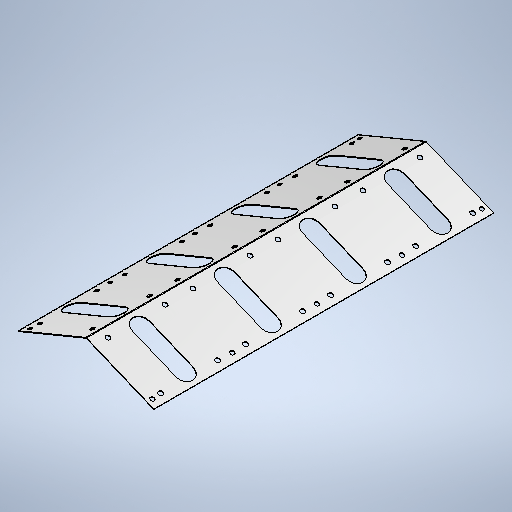
# Autodesk Inventor part: DMF 01 11 cylinder sheet cap v2.1
Saved by Autodesk Inventor 2026.2 (Build 302298010, 298A)
## iProperties
Created: 2024-04-28
Part Number: DMF 01 11 cylinder sheet cap v2.1
Material: Stainless Steel AISI 304
Document SubType Name: Sheet Metal
Designer: pokla
Density: 8 g/cm^3
Appearance: Chrome - Satin
Sheet Metal Rule: Default
Sheet Metal Width: 423,788 mm
Sheet Metal Length: 983,000 mm
Sheet Metal Area: 416583,808 mm^2
Flat Pattern Width: 42.3788 cm
Flat Pattern Length: 98.3 cm
Flat Pattern Area: 4165.84 cm^2
Stock Number: Барабан_Лист_Крышка
d192: 145,000 mm
d193: 50,000 mm
Author: pokla
Autodesk Inventor part; units mm, degrees
ref_plane "YZ Plane" through (0, 0, 0) normal (1, 0, 0) x (0, 1, 0)
ref_plane "XZ Plane" through (0, 0, 0) normal (0, 1, 0) x (-1, 0, 0)
ref_plane "XY Plane" through (0, 0, 0) normal (0, 0, 1) x (1, 0, 0)
sketch "Sketch1" plane through (0, 0, 0) normal (0, 0, 1) x (1, 0, 0)
  line L0 (-197.081968, 197.081968) -> (0, 278.715992) construction
  line L1 (0, 278.715992) -> (197.081968, 197.081968) construction
  line L2 (197.081968, 197.081968) -> (278.715992, 0) construction
  line L3 (278.715992, 0) -> (197.081968, -197.081968) construction
  line L4 (197.081968, -197.081968) -> (0, -278.715992) construction
  line L5 (0, -278.715992) -> (-197.081968, -197.081968) construction
  line L6 (-197.081968, -197.081968) -> (-278.715992, 0) construction
  line L7 (-278.715992, 0) -> (-197.081968, 197.081968) construction
  line L8 (1.530734, 278.081941) -> (196.250476, 197.426383)
  line L9 (-1.530734, 278.081941) -> (-196.250476, 197.426383)
  arc A0 (1.530734, 278.081941) -> (-1.530734, 278.081941) centre (0, 274.386423) ccw
  point P0 (0, 0)
  point P1 (0, 0)
  dimension "d46" = 515
  dimension "d47" = 0.9
  dimension "d48" = 4
  measures "d46" distance between parallel lines of L7 L3
  measures "d47" distance of L0.start L9.end
  measures "d48" radius of A0
contour flange "Contour Flange2" sketch "Sketch1" thickness 2 bend radius 2 width 983 along (0, 0, -1) mid plane no both sides no wall seen from (98.890605, 237.754162, 0) lies toward (-0.3826834, -0.9238795, 0) curves L8 A0 L9
bend "Bend4"
corner "Corner4"
sketch "Sketch14" plane through (1.530734, 278.081941, 0) normal (0.3826834, 0.9238795, 0) x (0.9238795, -0.3826834, 0)
  line L0 (173.881565, 148) -> (173.881565, 98) construction
  line L1 (173.881565, 98) -> (36.881565, 98)
  line L2 (36.881565, 98) -> (36.881565, 148) construction
  line L3 (36.881565, 148) -> (173.881565, 148)
  circle A0 centre (187.881565, 205.5) radius 6.5
  circle A1 centre (22.881565, 205.5) radius 6.5
  line L4 (105.381565, 98) -> (105.381565, 148) construction
  line L5 (210.76313, 0) -> (0, 0)
  line L6 (105.381565, 123) -> (173.881565, 123) construction
  circle A2 centre (22.881565, 40.5) radius 6.5
  circle A3 centre (187.881565, 40.5) radius 6.5
  arc A4 (173.881565, 98) -> (173.881565, 148) centre (173.881565, 123) ccw
  arc A5 (36.881565, 148) -> (36.881565, 98) centre (36.881565, 123) ccw
  point P0 (105.381565, 0)
  dimension "d163" = 13
  dimension "d164" = 137
  dimension "d165" = 50
  dimension "d167" = 165
  dimension "d171" = 98
  dimension "d181" = 165
  constraints: 12 end point, 6 centre point, 5 midpoint, 4 point on circle, 4 tangent, 2 parallel, 1 perpendicular, 1 vertical alignment, 3 other
  measures "d163" diameter of A0
  measures "d164" distance of L2.end L0.start
  measures "d165" distance of L0.start L0.end
  measures "d167" distance of A1.centre A0.centre
  measures "d171" distance between parallel lines of L5 L1
  measures "d181" distance of A1.centre A2.centre
extrude "Cut2" cut sketch "Sketch14" against normal through all
pattern_linear "Rectangular Pattern7" count 4 spacing 246 along (0, 0, -1) of "Cut2"
pattern_circular "Circular Pattern2" count 2 over 45 about axis through (0, 0, -10) along (0, 0, 1) of "Cut2", "Rectangular Pattern7"
sketch "Sketch16" plane through (0.765367, 276.234182, -983) normal (-0.3826834, -0.9238795, 0) x (0.9238795, -0.3826834, 0)
  circle A0 centre (189.76313, 968) radius 6
  line L0 (189.76313, 968) -> (189.76313, 15) construction
  circle A1 centre (189.76313, 15) radius 6
  circle A2 centre (189.76313, 246.5) radius 6
  circle A3 centre (189.76313, 491.5) radius 6
  circle A4 centre (189.76313, 736.5) radius 6
  line L1 (0, 983) -> (210.76313, 983)
  line L2 (210.76313, 983) -> (210.76313, 0)
  line L3 (210.76313, 983) -> (210.76313, 0)
  line L4 (210.76313, 0) -> (0, 0)
  line L5 (210.76313, 0) -> (0, 0)
  point P0 (105.003138, 983)
  dimension "d194" = 12
  dimension "d196" = 21
  dimension "d197" = 15
  dimension "d198" = 15
  dimension "d199" = 231.5
  dimension "d200" = 245
  dimension "d201" = 245
  dimension "d205" = 231.5
  constraints: 6 end point, 5 centre point, 4 equal radius, 2 point on line, 1 coincident, 1 midpoint, 1 vertical
  measures "d194" diameter of A0
  measures "d196" distance from line of L0.start L2
  measures "d197" distance from line of L1 L0.start
  measures "d198" distance from line of L0.end L4
  measures "d199" distance of L0.start A4.centre
  measures "d200" distance of A3.centre A4.centre
  measures "d201" distance of A3.centre A2.centre
  measures "d205" distance of A2.centre L0.end
extrude "Cut3" cut sketch "Sketch16" against normal blind 2
mirror "Mirror6" about plane through (0, 0, 0) normal (1, 0, 0) of "Cut3"
equation "\"d46\" = Барабан_размер_по_плоскостям"
equation "\"d47\" = Барабан_отступ_развертки"
equation "\"d48\" = BendRadius + Thickness"
equation "\"d49\" = Thickness"
equation "\"d50\" = BendReliefWidth"
equation "\"d51\" = BendReliefDepth"
equation "\"d52\" = MinimumRemnant"
equation "\"d53\" = TransitionRadius"
equation "\"d55\" = BendRadius"
equation "\"d57\" = CornerReliefSize"
equation "\"d58\" = GapSize"
equation "\"d59\" = JacobiRadiusSize"
equation "\"BendRadius\" = Thickness"
equation "\"BendReliefWidth\" = Thickness"
equation "\"BendReliefDepth\" = 0.5 * Thickness"
equation "\"CornerReliefSize\" = 4 * Thickness"
equation "\"MinimumRemnant\" = 2 * Thickness"
equation "\"TransitionRadius\" = BendRadius"
equation "\"JacobiRadiusSize\" = BendRadius"
equation "\"GapSize\" = Thickness"
equation "\"d192\" = 145"
equation "\"Барабан_размер_по_плоскостям\" = 515"
equation "\"Барабан_отступ_развертки\" = 0.9"
equation "\"Thickness\" = 2"
body "Solid2"
